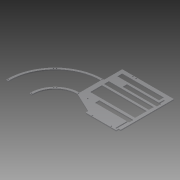
# Autodesk Inventor part: Runner Rails v2
Saved by Autodesk Inventor 2013 (Build 170138000, 138)
## iProperties
Created: 2013-01-15
Part Number: Runner Rails v2
Material: Polycarbonate, Clear
Document SubType Name: Modeling
Designer: actoennies
Mass: 484.62 g
Surface Area: 1702.19 cm^2
Volume: 403.85 cm^3
Density: 1.2 g/cm^3
Author: actoennies
Autodesk Inventor part; units mm, degrees
ref_plane "YZ Plane" through (0, 0, 0) normal (1, 0, 0) x (0, 1, 0)
ref_plane "XZ Plane" through (0, 0, 0) normal (0, 1, 0) x (-1, 0, 0)
ref_plane "XY Plane" through (0, 0, 0) normal (0, 0, 1) x (1, 0, 0)
sketch "Sketch1" plane through (0, 0, 0) normal (0, 1, 0) x (-1, 0, 0)
  arc A0 (0, -273.05) -> (273.05, 0) centre (0, 0) ccw
  arc A1 (0, -285.75) -> (285.75, 0) centre (0, 0) ccw
  arc A2 (0, -146.05) -> (146.05, 0) centre (0, 0) ccw
  arc A3 (0, -133.35) -> (133.35, 0) centre (0, 0) ccw
  line L0 (0, -285.75) -> (-6.35, -285.75)
  line L1 (146.05, 0) -> (146.05, 6.35)
  line L2 (133.35, 0) -> (133.35, 6.35)
  line L3 (273.05, 6.35) -> (273.05, 0)
  line L4 (285.75, 6.35) -> (285.75, 0)
  circle A4 centre (103.1708, -94.1906) radius 3.3782
  circle A5 centre (94.1906, -103.1708) radius 3.3782
  circle A6 centre (279.4, 0) radius 3.3782
  circle A7 centre (139.7, 0) radius 3.3782
  circle A8 centre (202.0047, -193.0245) radius 3.3782
  circle A9 centre (193.0245, -202.0047) radius 3.3782
  circle A10 centre (0, -279.4) radius 3.3782
  circle A11 centre (0, -139.7) radius 3.3782
  circle A12 centre (-55.2746, -139.7) radius 3.3782
  circle A13 centre (-78.3684, -279.4) radius 3.3782
  line L5 (285.75, 6.35) -> (273.05, 6.35)
  line L6 (146.05, 6.35) -> (133.35, 6.35)
  line L7 (-314.96, -285.75) -> (-314.96, -273.05)
  line L8 (-101.6, -133.35) -> (-127, -133.35)
  line L9 (-127, -146.05) -> (-101.6, -146.05)
  line L10 (-314.96, -146.05) -> (-314.96, -133.35)
  line L11 (-6.35, -285.75) -> (-6.35, -393.7)
  line L12 (-6.35, -393.7) -> (-314.325, -393.7)
  line L13 (-314.325, -393.7) -> (-314.325, -76.2)
  line L14 (-314.325, -76.2) -> (-120.65, -76.2)
  line L15 (-120.65, -76.2) -> (0, -133.35)
  line L16 (0, -285.75) -> (-6.35, -285.75)
  line L17 (0, -146.05) -> (0, -273.05)
  dimension "d10" = 12.7
  dimension "d11" = 12.7
  dimension "d13" = 12.7
  dimension "d14" = 6.7564
  dimension "d15" = 6.7564
  dimension "d16" = 6.7564
  dimension "d18" = 6.7564
  dimension "d20" = 6.35
  dimension "d21" = 6.7564
  dimension "d22" = 6.7564
  dimension "d23" = 6.7564
  dimension "d26" = 6.7564
  dimension "d30" = 6.7564
  dimension "d32" = 6.7564
  dimension "d66" = 25.4
  dimension "d67" = 0
  dimension "d72" = 12.7
  dimension "d81" = 107.95
  dimension "d82" = 133.35
  dimension "d83" = 279.4
  dimension "d84" = 6.35
  dimension "d85" = 317.5
  dimension "d86" = 193.675
  dimension "d87" = 55.2746
  dimension "d88" = 139.7
  dimension "d91" = 307.975
  constraints: 36 end point, 14 centre point, 9 point on circle, 4 perpendicular, 3 coincident, 2 collinear, 2 parallel, 2 tangent, 1 horizontal, 1 point on line, 1 vertical, 2 other
  measures "d10" distance between parallel lines of L1 L2
  measures "d11" distance between parallel lines of L3 L4
  measures "d13" distance of L9.end L8.start
  measures "d14" diameter of A4
  measures "d15" diameter of A5
  measures "d16" diameter of A6
  measures "d18" diameter of A7
  measures "d20" distance from line of L1 A7.centre
  measures "d21" diameter of A8
  measures "d22" diameter of A9
  measures "d23" diameter of A10
  measures "d26" diameter of A11
  measures "d30" diameter of A12
  measures "d32" diameter of A13
  measures "d66" distance of L8.start L8.end
  measures "d67" vertical distance of L8.end L8.start
  measures "d72" distance of L9.start L8.end
  measures "d81" distance of L0.end L11.end
  measures "d82" horizontal distance of L2.start A10.centre
  measures "d83" distance of A0.centre A10.centre
  measures "d84" distance from line of A10.centre L11
  measures "d85" distance of L12.end L13.end
  measures "d86" distance of L13.end L14.end
  measures "d87" distance of A11.centre A12.centre
  measures "d88" vertical distance of A1.centre A12.centre
  measures "d91" distance of L11.end L12.end
extrude "Extrusion7" add sketch "Sketch1" along normal blind 6.35
sketch "Sketch7" plane through (0, 0, 0) normal (0, -1, 0) x (1, 0, 0)
  line L0 (0, -273.05) -> (0, -146.05) projected
  line L1 (314.325, -76.2) -> (314.325, -393.7) projected
  line L2 (314.325, -234.95) -> (0, -234.95)
  line L3 (301.625, -139.7) -> (301.625, -165.1)
  line L4 (301.625, -165.1) -> (98.425, -165.1)
  line L5 (98.425, -165.1) -> (98.425, -139.7)
  line L6 (98.425, -139.7) -> (301.625, -139.7)
  line L7 (301.625, -330.2) -> (301.625, -304.8)
  line L8 (301.625, -304.8) -> (98.425, -304.8)
  line L9 (98.425, -304.8) -> (98.425, -330.2)
  line L10 (98.425, -330.2) -> (301.625, -330.2)
  dimension "d92" = 25.4
  dimension "d93" = 203.2
  dimension "d94" = 12.7
  dimension "d95" = 69.85
  constraints: 18 end point, 4 symmetric about line, 3 perpendicular, 2 parallel, 1 midpoint, 1 point on line
  measures "d92" distance of L3.start L3.end
  measures "d93" distance of L3.end L4.end
  measures "d94" distance between parallel lines of L1 L3
  measures "d95" distance between parallel lines of L2 L4
extrude "Extrusion8" cut sketch "Sketch7" against normal blind 6.35
sketch "Sketch8" plane through (0, 6.35, 0) normal (0, 1, 0) x (1, 0, 0)
  line L0 (98.425, 165.1) -> (301.625, 165.1) projected
  line L1 (301.625, 304.8) -> (98.425, 304.8) projected
  circle A0 centre (78.3684, 279.4) radius 3.3782 projected
  line L2 (314.325, 76.2) -> (314.325, 393.7) projected
  line L3 (314.325, 393.7) -> (6.35, 393.7) projected
  line L4 (0, 273.05) -> (0, 146.05) projected
  line L5 (295.275, 367.3082) -> (295.275, 342.9)
  line L6 (295.275, 342.9) -> (28.575, 342.9)
  line L7 (28.575, 342.9) -> (28.575, 371.475)
  line L8 (28.575, 371.475) -> (295.275, 371.475)
  line L9 (295.275, 371.475) -> (295.275, 367.3082)
  line L10 (295.275, 292.1) -> (28.575, 292.1)
  line L11 (28.575, 292.1) -> (28.575, 263.525)
  line L12 (28.575, 263.525) -> (295.275, 263.525)
  line L13 (295.275, 263.525) -> (295.275, 292.1)
  line L14 (295.275, 250.825) -> (28.575, 250.825)
  line L15 (28.575, 250.825) -> (28.575, 222.25)
  line L16 (28.575, 222.25) -> (295.275, 222.25)
  line L17 (295.275, 222.25) -> (295.275, 250.825)
  line L18 (295.275, 209.55) -> (295.275, 180.975)
  line L19 (295.275, 180.975) -> (28.575, 180.975)
  line L20 (28.575, 180.975) -> (28.575, 209.55)
  line L21 (28.575, 209.55) -> (295.275, 209.55)
  dimension "d100" = 90
  dimension "d101" = 22.225
  dimension "d102" = 19.05
  dimension "d103" = 28.575
  dimension "d104" = 266.7
  dimension "d105" = 28.575
  dimension "d106" = 19.05
  dimension "d107" = 12.7
  dimension "d108" = 266.7
  dimension "d109" = 28.575
  dimension "d110" = 28.575
  dimension "d111" = 12.7
  dimension "d112" = 12.7
  dimension "d113" = 266.7
  dimension "d114" = 19.05
  dimension "d115" = 19.05
  constraints: 34 end point, 7 parallel, 7 perpendicular, 2 collinear
  measures "d100" angle of L6 L7
  measures "d101" distance between parallel lines of L3 L8
  measures "d102" distance between parallel lines of L2 L5
  measures "d103" distance between parallel lines of L8 L6
  measures "d104" distance of L7.end L8.end
  measures "d105" distance of L10.end L11.end
  measures "d106" distance between parallel lines of L2 L13
  measures "d107" distance between parallel lines of L1 L10
  measures "d108" distance of L11.end L12.end
  measures "d109" distance of L14.end L15.end
  measures "d110" distance of L18.start L18.end
  measures "d111" distance between parallel lines of L12 L14
  measures "d112" distance between parallel lines of L21 L16
  measures "d113" distance between parallel lines of L20 L18
  measures "d114" distance between parallel lines of L2 L17
  measures "d115" distance between parallel lines of L2 L18
extrude "Extrusion9" cut sketch "Sketch8" against normal blind 25.4
sketch "Sketch9" plane through (0, 6.35, 0) normal (0, 1, 0) x (1, 0, 0)
  line L0 (314.325, 76.2) -> (314.325, 393.7) projected
  line L1 (295.275, 371.475) -> (295.275, 88.9)
  line L2 (295.275, 88.9) -> (288.925, 88.9)
  line L3 (288.925, 88.9) -> (288.925, 381)
  line L4 (288.925, 381) -> (295.275, 381)
  line L5 (295.275, 381) -> (295.275, 371.475)
  dimension "d118" = 282.575
  dimension "d119" = 6.35
  dimension "d120" = 292.1
  constraints: 10 end point, 2 parallel, 2 perpendicular, 1 collinear, 1 point on line
  measures "d118" distance of L1.start L1.end
  measures "d119" distance of L1.end L2.end
  measures "d120" distance of L2.end L3.end
extrude "Extrusion10" cut sketch "Sketch9" against normal blind 25.4
sketch "Sketch10" plane through (0, 6.35, 0) normal (0, 1, 0) x (1, 0, 0)
  line L0 (120.65, 76.2) -> (314.325, 76.2) projected
  line L1 (0, 273.05) -> (0, 146.05) projected
  line L2 (120.65, 76.2) -> (120.65, 63.5)
  line L3 (120.65, 63.5) -> (145.3457, 38.8043)
  line L4 (145.3457, 38.8043) -> (302.8387, 38.8043)
  line L5 (302.8387, 38.8043) -> (302.8387, 76.2)
  dimension "d123" = 12.7
  dimension "d124" = 34.925
  dimension "d125" = 135
  constraints: 8 end point, 2 perpendicular, 1 parallel, 1 point on line
  measures "d123" distance of L0.start L2.end
  measures "d124" distance of L2.end L3.end
  measures "d125" angle of L2 L3
extrude "Extrusion11" add sketch "Sketch10" against normal blind 6.35
sketch "Sketch13" plane through (0, 6.35, 0) normal (0, 1, 0) x (1, 0, 0)
  line L0 (288.925, 88.9) -> (288.925, 139.7) projected
  line L1 (288.925, 139.7) -> (98.425, 139.7) projected
  line L2 (288.925, 381) -> (295.275, 381) projected
  line L3 (295.275, 88.9) -> (288.925, 88.9) projected
  line L4 (145.3457, 38.8043) -> (302.8387, 38.8043) projected
  line L5 (302.8387, 38.8043) -> (302.8387, 76.2) projected
  line L6 (0, 273.05) -> (0, 146.05) projected
  line L7 (98.425, 127) -> (98.425, 101.6)
  line L8 (98.425, 101.6) -> (288.925, 101.6)
  line L9 (98.425, 127) -> (288.925, 127)
  line L10 (288.925, 88.9) -> (288.925, 44.45)
  line L11 (288.925, 44.45) -> (295.275, 44.45)
  line L12 (295.275, 44.45) -> (295.275, 88.9)
  dimension "d135" = 25.4
  dimension "d136" = 336.55
  dimension "d137" = 12.7
  constraints: 12 end point, 4 perpendicular, 2 parallel, 2 point on line
  measures "d135" distance of L7.start L7.end
  measures "d136" distance between parallel lines of L2 L11
  measures "d137" distance between parallel lines of L1 L9
extrude "Extrusion13" cut sketch "Sketch13" against normal blind 25.4
sketch "Sketch14" plane through (0, 6.35, 0) normal (0, 1, 0) x (1, 0, 0)
  line L0 (311.15, 79.375) -> (304.8, 79.375) projected
  line L1 (304.8, 79.375) -> (304.8, 85.725) projected
  line L2 (304.8, 85.725) -> (311.15, 85.725) projected
  line L3 (311.15, 85.725) -> (311.15, 79.375) projected
  line L4 (6.35, 381) -> (301.625, 381) projected
  line L5 (301.625, 381) -> (301.625, 76.2) projected
  line L6 (301.625, 76.2) -> (314.325, 76.2) projected
  line L7 (314.325, 76.2) -> (314.325, 393.7) projected
  line L8 (314.325, 393.7) -> (6.35, 393.7) projected
  line L9 (6.35, 393.7) -> (6.35, 381) projected
  line L10 (311.15, 390.525) -> (311.15, 384.175) projected
  line L11 (311.15, 384.175) -> (304.8, 384.175) projected
  line L12 (304.8, 384.175) -> (304.8, 390.525) projected
  line L13 (304.8, 390.525) -> (311.15, 390.525) projected
  line L14 (15.875, 384.175) -> (9.525, 384.175) projected
  line L15 (9.525, 384.175) -> (9.525, 390.525) projected
  line L16 (9.525, 390.525) -> (15.875, 390.525) projected
  line L17 (15.875, 390.525) -> (15.875, 384.175) projected
  line L18 (145.3457, 38.8043) -> (302.8387, 38.8043) projected
  line L19 (301.625, 139.7) -> (295.275, 139.7) projected
  line L20 (152.2186, 54.6793) -> (152.2186, 48.3293)
  line L21 (152.2186, 48.3293) -> (158.5686, 48.3293)
  line L22 (158.5686, 48.3293) -> (158.5686, 54.6793)
  line L23 (158.5686, 54.6793) -> (152.2186, 54.6793)
  dimension "d146" = 6.35
  dimension "d148" = 6.35
  dimension "d149" = 9.525
  constraints: 8 end point, 3 perpendicular, 1 parallel
  measures "d146" distance of L20.start L20.end
  measures "d148" distance of L20.end L21.end
  measures "d149" distance between parallel lines of L18 L21
extrude "Extrusion15" cut sketch "Sketch14" against normal blind 25.4 contours L23 L22 L21 L20
sketch "Sketch16" plane through (0, 6.35, 0) normal (0, 1, 0) x (1, 0, 0)
  line L0 (288.925, 165.1) -> (288.925, 180.975) projected
  line L1 (288.925, 209.55) -> (288.925, 222.25) projected
  line L2 (288.925, 250.825) -> (288.925, 263.525) projected
  line L3 (288.925, 292.1) -> (288.925, 304.8) projected
  line L4 (295.275, 304.8) -> (295.275, 165.1) projected
  line L5 (295.275, 165.1) -> (301.625, 165.1) projected
  line L6 (288.925, 165.1) -> (295.275, 165.1)
  line L7 (288.925, 180.975) -> (295.275, 180.975)
  line L8 (288.925, 222.25) -> (295.275, 222.25)
  line L9 (288.925, 209.55) -> (295.275, 209.55)
  line L10 (288.925, 304.8) -> (295.275, 304.8)
  line L11 (288.925, 292.1) -> (295.275, 292.1)
  line L12 (288.925, 263.525) -> (295.275, 263.525)
  line L13 (288.925, 250.825) -> (295.275, 250.825)
  constraints: 16 end point, 6 equal length, 6 point on line, 2 perpendicular
extrude "Extrusion16" add sketch "Sketch16" against normal blind 6.35
sketch "Sketch17" plane through (0, 6.35, 0) normal (0, 1, 0) x (1, 0, 0)
  line L0 (288.925, 44.45) -> (288.925, 101.6) projected
  line L1 (288.925, 101.6) -> (98.425, 101.6) projected
  line L2 (98.425, 127) -> (288.925, 127) projected
  line L3 (288.925, 342.9) -> (28.575, 342.9) projected
  line L4 (28.575, 371.475) -> (288.925, 371.475) projected
  line L5 (288.925, 127) -> (288.925, 101.6)
  line L6 (276.225, 127) -> (276.225, 101.6)
  line L7 (288.925, 342.9) -> (288.925, 371.475)
  line L8 (276.225, 371.475) -> (276.225, 342.9)
  dimension "d155" = 12.7
  dimension "d156" = 12.7
  constraints: 8 end point, 4 point on line, 3 parallel, 1 collinear
  measures "d155" distance between parallel lines of L6 L5
  measures "d156" distance between parallel lines of L7 L8
extrude "Extrusion17" add sketch "Sketch17" against normal blind 6.35
sketch "Sketch18" plane through (0, 6.35, 0) normal (0, 1, 0) x (1, 0, 0)
  line L0 (288.925, 44.45) -> (288.925, 139.7) projected
  line L1 (295.275, 139.7) -> (295.275, 44.45) projected
  line L2 (295.275, 44.45) -> (288.925, 44.45) projected
  line L3 (145.3457, 38.8043) -> (302.8387, 38.8043) projected
  line L4 (295.275, 70.5543) -> (288.925, 70.5543)
  dimension "d159" = 31.75
  constraints: 2 end point, 2 point on line, 1 perpendicular
  measures "d159" distance between parallel lines of L3 L4
extrude "Extrusion18" add sketch "Sketch18" against normal blind 6.35
sketch "Sketch19" plane through (0, 6.35, 0) normal (0, 1, 0) x (1, 0, 0)
  line L0 (314.325, 393.7) -> (6.35, 393.7) projected
  line L1 (6.35, 393.7) -> (6.35, 285.75) projected
  circle A0 centre (76.2, 387.35) radius 3.3782
  dimension "d162" = 6.7564
  dimension "d164" = 6.35
  dimension "d165" = 69.85
  constraints: 1 centre point
  measures "d162" diameter of A0
  measures "d164" distance from line of L0 A0.centre
  measures "d165" distance from line of L1 A0.centre
extrude "Extrusion19" cut sketch "Sketch19" against normal blind 25.4
sketch "Sketch20" plane through (0, 6.35, 0) normal (0, 1, 0) x (1, 0, 0)
  circle A0 centre (95.25, 387.35) radius 3.3782 projected
extrude "Extrusion20" cut sketch "Sketch20" against normal blind 25.4
sketch "Sketch21" plane through (0, 6.35, 0) normal (0, 1, 0) x (1, 0, 0)
  line L0 (158.5686, 54.6793) -> (158.5686, 48.3293) projected
  line L1 (145.3457, 38.8043) -> (302.8387, 38.8043) projected
  line L2 (302.8387, 38.8043) -> (302.8387, 76.2) projected
  circle A0 centre (155.3936, 67.3793) radius 3.3782
  circle A1 centre (267.9137, 67.3793) radius 3.3782
  dimension "d170" = 6.7564
  dimension "d171" = 6.7564
  dimension "d172" = 28.575
  dimension "d173" = 34.925
  dimension "d174" = 28.575
  dimension "d176" = 3.175
  constraints: 2 centre point
  measures "d170" diameter of A0
  measures "d171" diameter of A1
  measures "d172" distance from line of L1 A1.centre
  measures "d173" distance from line of L2 A1.centre
  measures "d174" distance from line of L1 A0.centre
  measures "d176" distance from line of A0.centre L0
extrude "Extrusion21" cut sketch "Sketch21" against normal blind 25.4
sketch "Sketch22" plane through (0, 6.35, 0) normal (0, 1, 0) x (1, 0, 0)
  line L0 (288.925, 330.2) -> (288.925, 381) projected
  line L1 (288.925, 381) -> (295.275, 381) projected
  line L2 (295.275, 381) -> (295.275, 330.2) projected
  line L3 (288.925, 358.775) -> (295.275, 358.775)
  dimension "d179" = 22.225
  constraints: 2 end point, 2 point on line, 1 perpendicular
  measures "d179" distance between parallel lines of L1 L3
extrude "Extrusion22" add sketch "Sketch22" against normal blind 6.35
sketch "Sketch23" plane through (0, 6.35, 0) normal (0, 1, 0) x (1, 0, 0)
  line L0 (158.5686, 48.3293) -> (152.2186, 48.3293) projected
  line L1 (152.2186, 48.3293) -> (152.2186, 54.6793) projected
  line L2 (152.2186, 54.6793) -> (158.5686, 54.6793) projected
  line L3 (158.5686, 54.6793) -> (158.5686, 48.3293) projected
  line L4 (120.65, 63.5) -> (145.3457, 38.8043) projected
  line L5 (145.3457, 38.8043) -> (302.8387, 38.8043) projected
  line L6 (302.8387, 38.8043) -> (302.8387, 76.2) projected
  line L7 (28.575, 371.475) -> (276.225, 371.475) projected
  line L8 (302.8387, 61.0293) -> (123.1207, 61.0293)
  dimension "d182" = 22.225
  constraints: 2 end point, 2 point on line, 1 parallel
  measures "d182" distance between parallel lines of L5 L8
extrude "Extrusion23" cut sketch "Sketch23" against normal blind 6.35
sketch "Sketch24" plane through (0, 6.35, 0) normal (0, 1, 0) x (1, 0, 0)
  line L0 (276.225, 127) -> (276.225, 101.6) projected
  line L1 (276.225, 101.6) -> (98.425, 101.6) projected
  line L2 (98.425, 101.6) -> (98.425, 127) projected
  line L3 (98.425, 127) -> (276.225, 127) projected
extrude "Extrusion24" add sketch "Sketch24" against normal blind 6.35
sketch "Sketch25" plane through (0, 6.35, 0) normal (0, 1, 0) x (1, 0, 0)
  line L0 (295.275, 222.25) -> (28.575, 222.25) projected
  line L1 (295.275, 209.55) -> (295.275, 180.975) projected
  line L2 (28.575, 209.55) -> (295.275, 209.55) projected
  line L3 (295.275, 70.5543) -> (288.925, 70.5543) projected
  line L4 (28.575, 209.55) -> (28.575, 222.25)
  line L5 (295.275, 222.25) -> (295.275, 209.55)
  constraints: 4 end point, 1 collinear, 1 perpendicular
extrude "Extrusion25" cut sketch "Sketch25" against normal blind 25.4
body "Solid2"
